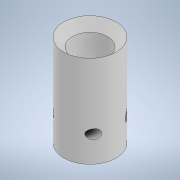
# Autodesk Inventor part: catch vertical seal-tighttol-thread
Saved by Autodesk Inventor 2020 (Build 240168000, 168)
## iProperties
Created: 2022-01-16
Part Number: catch vertical seal-tighttol-thread
Material: Generic
Document SubType Name: Modeling
Designer: pab2
Density: 1 g/cm^3
Appearance: Default
Author: pab2
Autodesk Inventor part; units mm, degrees
ref_plane "YZ Plane" through (0, 0, 0) normal (1, 0, 0) x (0, 1, 0)
ref_plane "XZ Plane" through (0, 0, 0) normal (0, 1, 0) x (-1, 0, 0)
ref_plane "XY Plane" through (0, 0, 0) normal (0, 0, 1) x (1, 0, 0)
sketch "Sketch1" plane through (0, 0, 0) normal (0, 0, 1) x (1, 0, 0)
  line L0 (0, 0) -> (6.223, 0)
  line L1 (0, 0) -> (6.223, 0) construction
  line L2 (6.223, 0) -> (6.223, 38.1)
  line L3 (0, 0) -> (0.762, 0)
  line L4 (0.762, 0) -> (0.762, 8.255)
  line L5 (0.762, 8.255) -> (6.223, 28.635729)
  line L6 (6.223, 28.635729) -> (6.223, 38.1)
  line L7 (0, 0) -> (12.7, 0)
  line L8 (0, -8.9154) -> (0, 53.4924)
  line L9 (6.223, 38.1) -> (12.20332, 44.08032)
  line L10 (6.223, 38.1) -> (14.68045, 38.1) construction
  line L11 (12.20332, 44.08032) -> (12.7, 0)
  line L12 (12.7, 0) -> (12.7, 44.577)
  line L13 (12.7, 44.577) -> (6.223, 38.1)
  line L14 (6.223, 38.1) -> (0, 38.1)
  line L15 (0, 8.255) -> (0.762, 8.255)
  line L16 (0, 8.255) -> (0, 38.1)
  line L17 (6.223, 28.635729) -> (0, 28.635729)
  line L18 (0, 28.635729) -> (8.60425, 28.635729)
  line L19 (8.60425, 28.635729) -> (0.762, 8.255)
  line L20 (8.60425, 28.635729) -> (8.60425, 40.48125)
  dimension "d0" = 6.223
  dimension "d1" = 0
  dimension "d2" = 38.1
  dimension "d3" = 90
  dimension "d4" = 0.762
  dimension "d5" = 8.255
  dimension "d6" = 165
  dimension "d7" = 12.7
  dimension "d18" = 45
  dimension "d58" = 8.60425
  constraints: 40 end point, 7 point on line, 4 horizontal, 4 perpendicular, 3 collinear, 2 equal length, 2 vertical, 1 parallel
  measures "d0" distance of L0.start L0.end
  measures "d1" distance between parallel lines of L0 L1
  measures "d2" distance of L0.end L2.end
  measures "d3" angle of L2 L0
  measures "d4" distance of L0.start L3.end
  measures "d5" distance of L3.end L4.end
  measures "d6" angle of L4 L5
  measures "d7" distance of L0.start L7.end
  measures "d18" angle of L10 L9
  measures "d58" distance of L17.end L18.end
sketch "Sketch1 outline for Revolution1" plane through (0, 0, 0) normal (0, 0, 1) x (1, 0, 0)
  line L0 (8.60425, 40.48125) -> (8.60425, 28.635729)
  line L1 (8.60425, 28.635729) -> (0.762, 8.255)
  line L2 (0.762, 8.255) -> (0.762, 0)
  line L3 (0.762, 0) -> (12.7, 0)
  line L4 (12.7, 0) -> (12.7, 44.577)
  line L5 (12.7, 44.577) -> (8.60425, 40.48125)
revolve "Revolution1" add sketch "Sketch1 outline for Revolution1" angle 360 about axis through (0, -10, 0) along (0, 1, 0)
sketch "Sketch3" plane through (0, 0, 0) normal (0, -1, 0) x (1, 0, 0)
  point P0 (0, 0)
  point P1 (0, 0)
  constraints: 1 coincident
hole "Hole2" at (0, 0, 0) direction (0, 1, 0) diameter 5.3594 depth 6.35 thread size "1/4-28 UNF" class "2B" standard "ANSI Unified Screw Threads"
sketch "Sketch4" plane through (0, 0, 0) normal (1, 0, 0) x (0, 1, 0)
  line L0 (0, 12.7) -> (0, -12.7) projected
  line L1 (0, 12.7) -> (0, 7.9248)
  line L2 (0, 7.9248) -> (12.7, 7.9248)
  line L3 (0, -12.7) -> (0, -7.9248)
  line L4 (0, -7.9248) -> (12.7, -7.9248)
  point P0 (0, 0)
  dimension "d28" = 4.7752
  dimension "d29" = 12.7
  dimension "d30" = 4.7752
  dimension "d31" = 12.7
  dimension "d32" = 90
  constraints: 8 end point, 2 perpendicular, 2 point on line
  measures "d28" distance of L0.start L1.end
  measures "d29" distance of L1.end L2.end
  measures "d30" distance of L0.end L3.end
  measures "d31" distance of L3.end L4.end
  measures "d32" angle of L3 L4
hole "Hole3" at (0, 12.7, 7.9248) at (0, 12.7, -7.9248) direction (-1, 0, 0) diameter 4.4958 end through all clearance for "Socket Head Cap Screw" size "#8" standard "Ansi Unified Screw Threads"
mirror "Mirror1" about plane through (0, 0, 0) normal (1, 0, 0) of "Hole3"
equation "\"d47\" = 55deg"
equation "\"Sketch5_Pitch\" = 0.90714"
body "Solid1"
